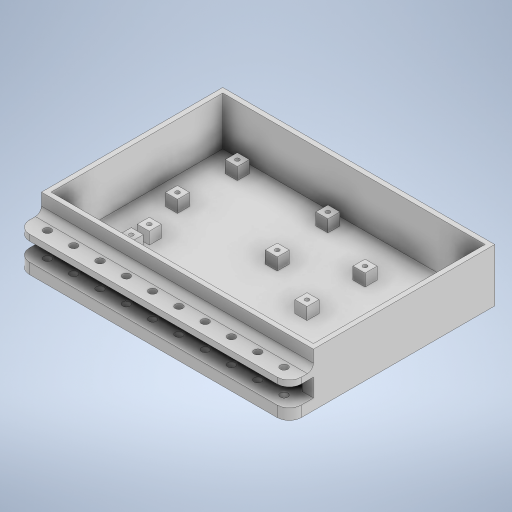
# Autodesk Inventor part: ebox
Saved by Autodesk Inventor 2024.3 (Build 283343000, 343)
## iProperties
Created: 2025-01-01
Part Number: ebox
Material: Generic
Document SubType Name: Modeling
Designer: email
Density: 1 g/cm^3
Appearance: Default
Author: email
Autodesk Inventor part; units mm, degrees
ref_plane "YZ Plane" through (0, 0, 0) normal (1, 0, 0) x (0, 1, 0)
ref_plane "XZ Plane" through (0, 0, 0) normal (0, 1, 0) x (-1, 0, 0)
ref_plane "XY Plane" through (0, 0, 0) normal (0, 0, 1) x (1, 0, 0)
sketch "Sketch1" plane through (0, 0, 0) normal (0, 1, 0) x (-1, 0, 0)
  line L0 (0, 0) -> (-225, 0)
  line L1 (-225, 0) -> (-225, -150)
  line L2 (-225, -150) -> (0, -150)
  line L3 (0, -150) -> (0, 0)
  line L4 (-12.5, -136.845) -> (-114.1, -136.845)
  line L5 (-114.1, -136.845) -> (-114.1, -83.505)
  line L6 (-114.1, -83.505) -> (-12.5, -83.505)
  line L7 (-12.5, -83.505) -> (-12.5, -136.845)
  line L8 (-4, -4) -> (-221, -4)
  line L9 (-221, -4) -> (-221, -146)
  line L10 (-221, -146) -> (-4, -146)
  line L11 (-4, -146) -> (-4, -4)
  line L12 (-153.3391, -114.3444) -> (-208.3391, -114.3444)
  line L13 (-208.3391, -114.3444) -> (-208.3391, -59.3444)
  line L14 (-208.3391, -59.3444) -> (-153.3391, -59.3444)
  line L15 (-153.3391, -59.3444) -> (-153.3391, -114.3444)
  line L16 (-12.6469, -54.1694) -> (-42.6469, -54.1694)
  line L17 (-42.6469, -54.1694) -> (-42.6469, -34.1694)
  line L18 (-42.6469, -34.1694) -> (-12.6469, -34.1694)
  line L19 (-12.6469, -34.1694) -> (-12.6469, -54.1694)
  line L20 (-15.41, -128.945) -> (-4, -128.945)
  line L21 (-4, -128.945) -> (-4, -117.045)
  line L22 (-4, -117.045) -> (-15.41, -117.045)
  line L23 (-15.41, -117.045) -> (-15.41, -128.945)
  circle A0 centre (-27.74, -134.305) radius 1.75
  circle A1 centre (-26.47, -86.045) radius 1.75
  circle A2 centre (-102.67, -134.305) radius 1.75
  circle A3 centre (-109.02, -86.045) radius 1.75
  circle A4 centre (-156.8391, -110.8444) radius 1.75
  circle A5 centre (-204.8391, -110.8444) radius 1.75
  circle A6 centre (-156.8391, -62.8444) radius 1.75
  circle A7 centre (-204.8391, -62.8444) radius 1.75
  circle A8 centre (-37.5669, -51.6294) radius 1.75
  circle A9 centre (-37.5669, -36.7094) radius 1.75
  line L24 (-22.74, -139.305) -> (-32.74, -139.305)
  line L25 (-32.74, -139.305) -> (-32.74, -129.305)
  line L26 (-32.74, -129.305) -> (-22.74, -129.305)
  line L27 (-22.74, -129.305) -> (-22.74, -139.305)
  line L28 (-22.74, -139.305) -> (-32.74, -129.305) construction
  line L29 (-32.74, -139.305) -> (-22.74, -129.305) construction
  line L30 (-21.47, -81.045) -> (-31.47, -81.045)
  line L31 (-31.47, -81.045) -> (-31.47, -91.045)
  line L32 (-31.47, -91.045) -> (-21.47, -91.045)
  line L33 (-21.47, -91.045) -> (-21.47, -81.045)
  line L34 (-21.47, -81.045) -> (-31.47, -91.045) construction
  line L35 (-31.47, -81.045) -> (-21.47, -91.045) construction
  line L36 (-114.02, -81.045) -> (-104.02, -81.045)
  line L37 (-104.02, -81.045) -> (-104.02, -91.045)
  line L38 (-104.02, -91.045) -> (-114.02, -91.045)
  line L39 (-114.02, -91.045) -> (-114.02, -81.045)
  line L40 (-114.02, -81.045) -> (-104.02, -91.045) construction
  line L41 (-104.02, -81.045) -> (-114.02, -91.045) construction
  line L42 (-107.67, -139.305) -> (-97.67, -139.305)
  line L43 (-97.67, -139.305) -> (-97.67, -129.305)
  line L44 (-97.67, -129.305) -> (-107.67, -129.305)
  line L45 (-107.67, -129.305) -> (-107.67, -139.305)
  line L46 (-107.67, -139.305) -> (-97.67, -129.305) construction
  line L47 (-97.67, -139.305) -> (-107.67, -129.305) construction
  line L48 (-151.8391, -115.8444) -> (-161.8391, -115.8444)
  line L49 (-161.8391, -115.8444) -> (-161.8391, -105.8444)
  line L50 (-161.8391, -105.8444) -> (-151.8391, -105.8444)
  line L51 (-151.8391, -105.8444) -> (-151.8391, -115.8444)
  line L52 (-151.8391, -115.8444) -> (-161.8391, -105.8444) construction
  line L53 (-161.8391, -115.8444) -> (-151.8391, -105.8444) construction
  line L54 (-209.8391, -115.8444) -> (-199.8391, -115.8444)
  line L55 (-199.8391, -115.8444) -> (-199.8391, -105.8444)
  line L56 (-199.8391, -105.8444) -> (-209.8391, -105.8444)
  line L57 (-209.8391, -105.8444) -> (-209.8391, -115.8444)
  line L58 (-209.8391, -115.8444) -> (-199.8391, -105.8444) construction
  line L59 (-199.8391, -115.8444) -> (-209.8391, -105.8444) construction
  line L60 (-209.8391, -57.8444) -> (-199.8391, -57.8444)
  line L61 (-199.8391, -57.8444) -> (-199.8391, -67.8444)
  line L62 (-199.8391, -67.8444) -> (-209.8391, -67.8444)
  line L63 (-209.8391, -67.8444) -> (-209.8391, -57.8444)
  line L64 (-209.8391, -57.8444) -> (-199.8391, -67.8444) construction
  line L65 (-199.8391, -57.8444) -> (-209.8391, -67.8444) construction
  line L66 (-161.8391, -57.8444) -> (-151.8391, -57.8444)
  line L67 (-151.8391, -57.8444) -> (-151.8391, -67.8444)
  line L68 (-151.8391, -67.8444) -> (-161.8391, -67.8444)
  line L69 (-161.8391, -67.8444) -> (-161.8391, -57.8444)
  line L70 (-161.8391, -57.8444) -> (-151.8391, -67.8444) construction
  line L71 (-151.8391, -57.8444) -> (-161.8391, -67.8444) construction
  line L72 (-42.5669, -46.6294) -> (-32.5669, -46.6294)
  line L73 (-32.5669, -46.6294) -> (-32.5669, -56.6294)
  line L74 (-32.5669, -56.6294) -> (-42.5669, -56.6294)
  line L75 (-42.5669, -56.6294) -> (-42.5669, -46.6294)
  line L76 (-42.5669, -46.6294) -> (-32.5669, -56.6294) construction
  line L77 (-32.5669, -46.6294) -> (-42.5669, -56.6294) construction
  line L78 (-32.5669, -41.7094) -> (-42.5669, -41.7094)
  line L79 (-42.5669, -41.7094) -> (-42.5669, -31.7094)
  line L80 (-42.5669, -31.7094) -> (-32.5669, -31.7094)
  line L81 (-32.5669, -31.7094) -> (-32.5669, -41.7094)
  line L82 (-32.5669, -41.7094) -> (-42.5669, -31.7094) construction
  line L83 (-42.5669, -41.7094) -> (-32.5669, -31.7094) construction
  line L84 (0, -4) -> (-225, -4)
  line L85 (-225, -4) -> (-225, 20)
  line L86 (-225, 20) -> (0, 20)
  line L87 (0, 20) -> (0, -4)
  circle A10 centre (-15, 10) radius 3.125
  circle A11 centre (-36.75, 10) radius 3.125
  circle A12 centre (-58.5, 10) radius 3.125
  circle A13 centre (-80.25, 10) radius 3.125
  circle A14 centre (-102, 10) radius 3.125
  circle A15 centre (-123.75, 10) radius 3.125
  circle A16 centre (-145.5, 10) radius 3.125
  circle A17 centre (-167.25, 10) radius 3.125
  circle A18 centre (-189, 10) radius 3.125
  circle A19 centre (-210.75, 10) radius 3.125
  point P0 (-156.8391, -62.8444)
  dimension "d0" = 225
  dimension "d1" = 150
  dimension "d2" = 101.6
  dimension "d3" = 53.34
  dimension "d5" = 4
  dimension "d6" = 217
  dimension "d7" = 142
  dimension "d8" = 4
  dimension "d9" = 8.5
  dimension "d10" = 55
  dimension "d11" = 55
  dimension "d12" = 30
  dimension "d13" = 20
  dimension "d14" = 7.9
  dimension "d15" = 8.5
  dimension "d16" = 11.9
  dimension "d17" = 2.54
  dimension "d18" = 3.5
  dimension "d19" = 15.24
  dimension "d20" = 3.5
  dimension "d21" = 3.5
  dimension "d22" = 3.5
  dimension "d23" = 2.54
  dimension "d24" = 13.97
  dimension "d26" = 2.54
  dimension "d27" = 90.17
  dimension "d28" = 2.54
  dimension "d29" = 96.52
  dimension "d30" = 3.5
  dimension "d31" = 3.5
  dimension "d32" = 3.5
  dimension "d33" = 3.5
  dimension "d34" = 3.5
  dimension "d35" = 3.5
  dimension "d36" = 3.5
  dimension "d38" = 3.5
  dimension "d39" = 3.5
  dimension "d40" = 3.5
  dimension "d41" = 3.5
  dimension "d42" = 3.5
  dimension "d43" = 3.5
  dimension "d44" = 2.54
  dimension "d45" = 5.08
  dimension "d46" = 5.08
  dimension "d47" = 2.54
  dimension "d54" = 10
  dimension "d55" = 10
  dimension "d56" = 10
  dimension "d57" = 10
  dimension "d58" = 10
  dimension "d59" = 10
  dimension "d60" = 10
  dimension "d61" = 10
  dimension "d65" = 10
  dimension "d66" = 10
  dimension "d67" = 10
  dimension "d68" = 10
  dimension "d69" = 10
  dimension "d70" = 10
  dimension "d71" = 10
  dimension "d72" = 10
  dimension "d73" = 10
  dimension "d74" = 10
  dimension "d75" = 10
  constraints: 176 end point, 34 parallel, 21 midpoint, 20 centre point, 18 horizontal, 17 perpendicular, 2 point on line, 18 other
  measures "d0" distance of L1.end L2.end
  measures "d1" distance of L0.end L1.end
  measures "d2" distance of L4.start L4.end
  measures "d3" distance of L4.end L5.end
  measures "d5" distance between parallel lines of L0 L8
  measures "d6" distance of L9.end L10.end
  measures "d7" distance of L8.end L9.end
  measures "d8" distance between parallel lines of L3 L11
  measures "d9" distance between parallel lines of L11 L7
  measures "d10" distance of L12.end L13.end
  measures "d11" distance of L13.end L14.end
  measures "d12" distance of L16.start L16.end
  measures "d13" distance of L16.end L17.end
  measures "d14" distance between parallel lines of L4 L20
  measures "d15" distance between parallel lines of L7 L21
  measures "d16" distance of L22.end L20.start
  measures "d17" distance from line of L4 A0.centre
  measures "d18" diameter of A0
  measures "d19" distance from line of L7 A0.centre
  measures "d20" diameter of A1
  measures "d21" diameter of A3
  measures "d22" diameter of A2
  measures "d23" distance from line of L6 A1.centre
  measures "d24" distance from line of L7 A1.centre
  measures "d26" distance from line of L4 A2.centre
  measures "d27" distance from line of A2.centre L7
  measures "d28" distance from line of L6 A3.centre
  measures "d29" distance from line of L7 A3.centre
  measures "d30" diameter of A4
  measures "d31" diameter of A5
  measures "d32" diameter of A6
  measures "d33" diameter of A7
  measures "d34" distance from line of L12 A4.centre
  measures "d35" distance from line of L15 A4.centre
  measures "d36" distance from line of L14 A6.centre
  measures "d38" distance from line of L13 A7.centre
  measures "d39" distance from line of L14 A7.centre
  measures "d40" distance from line of L13 A5.centre
  measures "d41" distance from line of L12 A5.centre
  measures "d42" diameter of A8
  measures "d43" diameter of A9
  measures "d44" distance from line of L16 A8.centre
  measures "d45" distance from line of L17 A8.centre
  measures "d46" distance from line of L17 A9.centre
  measures "d47" distance from line of L18 A9.centre
  measures "d54" distance of L24.end L25.end
  measures "d55" distance of L25.end L26.end
  measures "d56" distance of L42.end L43.end
  measures "d57" distance of L43.end L44.end
  measures "d58" distance of L31.end L32.end
  measures "d59" distance of L30.end L31.end
  measures "d60" distance of L37.end L38.end
  measures "d61" distance of L36.end L37.end
  measures "d65" distance of L48.end L49.end
  measures "d66" distance of L49.end L50.end
  measures "d67" distance of L54.end L55.end
  measures "d68" distance of L55.end L56.end
  measures "d69" distance of L66.end L67.end
  measures "d70" distance of L66.start L66.end
  measures "d71" distance of L62.end L60.start
  measures "d72" distance of L60.start L60.end
  measures "d73" distance of L73.end L74.end
  measures "d74" distance of L72.end L73.end
  measures "d75" distance of L78.start L78.end
extrude "Extrusion1" add sketch "Sketch1" against normal blind 4 contours L3 L84 L8 L1 L0 | L3 L2 L1 L84 L9 L10 L11 | L11 L22 L7 L6 L33 L30 L31 L37 L36 L39 L5 L4 L45 L42 L43 L25 L24 L27 L20 L10 L9 L8 | L11 L20 L7 L22 | L22 L23 L20 L7 L4 L27 L26 L25 L43 L44 L45 L5 L6 L39 L38 L37 L31 L32 L33 | L7 L20 L23 L22 | L33 L32 L31 L6 | L6 L31 L30 L33 | L27 L24 L25 L4 | L4 L25 L26 L27 | L37 L38 L39 L6 | L6 L39 L36 L37 | L43 L42 L45 L4 | L4 L45 L44 L43 | L15 L50 L51 L48 L49 L12 | L12 L49 L50 L15 | L12 L55 L56 L13 L62 L61 L14 L69 L68 L15 L50 L49 | L55 L54 L57 L56 L13 L12 | L12 L13 L56 L55 | L68 L69 L14 L15 | L15 L14 L69 L66 L67 L68 | L62 L63 L60 L61 L14 L13 | L13 L14 L61 L62 | L16 L73 L72 L75 L17 L18 L79 L78 L81 L19 | L73 L74 L75 L16 | L16 L75 L72 L73 | L81 L78 L79 L18 | L18 L79 L80 L81 | A0 | A1 | A2 | A3 | A4 | A5 | A6 | A7 | A8 | A9
extrude "Extrusion2" add sketch "Sketch1" along normal blind 40 contours L3 L84 L8 L1 L0 | L3 L2 L1 L84 L9 L10 L11
extrude "Extrusion3" add sketch "Sketch1" along normal blind 10 contours L33 L32 L31 L6 | L6 L31 L30 L33 | L27 L24 L25 L4 | L4 L25 L26 L27 | L37 L38 L39 L6 | L6 L39 L36 L37 | L43 L42 L45 L4 | L4 L45 L44 L43 | L15 L50 L51 L48 L49 L12 | L12 L49 L50 L15 | L55 L54 L57 L56 L13 L12 | L12 L13 L56 L55 | L68 L69 L14 L15 | L15 L14 L69 L66 L67 L68 | L62 L63 L60 L61 L14 L13 | L13 L14 L61 L62 | L73 L74 L75 L16 | L16 L75 L72 L73 | L81 L78 L79 L18 | L18 L79 L80 L81
extrude "Extrusion4" add sketch "Sketch1" along normal blind 5 and the other way blind 4 contours L0 L85 L86 L87
sketch "Sketch2" plane through (0, 40, 0) normal (0, 0, 1) x (1, 0, 0)
  line L0 (10, -20) -> (20, -20)
  line L1 (20, -20) -> (20, -35)
  line L2 (20, -35) -> (10, -35)
  line L3 (10, -35) -> (10, -20)
  line L4 (10, -20) -> (20, -35) construction
  line L5 (20, -20) -> (10, -35) construction
  line L6 (31.75, -20) -> (41.75, -20)
  line L7 (41.75, -20) -> (41.75, -35)
  line L8 (41.75, -35) -> (31.75, -35)
  line L9 (31.75, -35) -> (31.75, -20)
  line L10 (31.75, -20) -> (41.75, -35) construction
  line L11 (41.75, -20) -> (31.75, -35) construction
  line L12 (53.5, -20) -> (63.5, -20)
  line L13 (63.5, -20) -> (63.5, -35)
  line L14 (63.5, -35) -> (53.5, -35)
  line L15 (53.5, -35) -> (53.5, -20)
  line L16 (53.5, -20) -> (63.5, -35) construction
  line L17 (63.5, -20) -> (53.5, -35) construction
  line L18 (75.25, -20) -> (85.25, -20)
  line L19 (85.25, -20) -> (85.25, -35)
  line L20 (85.25, -35) -> (75.25, -35)
  line L21 (75.25, -35) -> (75.25, -20)
  line L22 (75.25, -20) -> (85.25, -35) construction
  line L23 (85.25, -20) -> (75.25, -35) construction
  line L24 (97, -20) -> (107, -20)
  line L25 (107, -20) -> (107, -35)
  line L26 (107, -35) -> (97, -35)
  line L27 (97, -35) -> (97, -20)
  line L28 (97, -20) -> (107, -35) construction
  line L29 (107, -20) -> (97, -35) construction
  line L30 (118.75, -20) -> (128.75, -20)
  line L31 (128.75, -20) -> (128.75, -35)
  line L32 (128.75, -35) -> (118.75, -35)
  line L33 (118.75, -35) -> (118.75, -20)
  line L34 (118.75, -20) -> (128.75, -35) construction
  line L35 (128.75, -20) -> (118.75, -35) construction
  line L36 (140.5, -20) -> (150.5, -20)
  line L37 (150.5, -20) -> (150.5, -35)
  line L38 (150.5, -35) -> (140.5, -35)
  line L39 (140.5, -35) -> (140.5, -20)
  line L40 (140.5, -20) -> (150.5, -35) construction
  line L41 (150.5, -20) -> (140.5, -35) construction
  line L42 (162.25, -20) -> (172.25, -20)
  line L43 (172.25, -20) -> (172.25, -35)
  line L44 (172.25, -35) -> (162.25, -35)
  line L45 (162.25, -35) -> (162.25, -20)
  line L46 (162.25, -20) -> (172.25, -35) construction
  line L47 (172.25, -20) -> (162.25, -35) construction
  line L48 (184, -20) -> (194, -20)
  line L49 (194, -20) -> (194, -35)
  line L50 (194, -35) -> (184, -35)
  line L51 (184, -35) -> (184, -20)
  line L52 (184, -20) -> (194, -35) construction
  line L53 (194, -20) -> (184, -35) construction
  line L54 (205.75, -20) -> (215.75, -20)
  line L55 (215.75, -20) -> (215.75, -35)
  line L56 (215.75, -35) -> (205.75, -35)
  line L57 (205.75, -35) -> (205.75, -20)
  line L58 (205.75, -20) -> (215.75, -35) construction
  line L59 (215.75, -20) -> (205.75, -35) construction
  line L60 (0, -35) -> (0, 0) projected
  line L61 (0, -35) -> (225, -35) projected
  point P0 (15, -27.5)
  point P1 (36.75, -27.5)
  point P2 (58.5, -27.5)
  point P3 (80.25, -27.5)
  point P4 (102, -27.5)
  point P5 (123.75, -27.5)
  point P6 (145.5, -27.5)
  point P7 (167.25, -27.5)
  point P8 (189, -27.5)
  point P9 (210.75, -27.5)
  dimension "d105" = 10
  dimension "d106" = 15
  dimension "d109" = 21.75
  dimension "d132" = 15
  dimension "d133" = 7.5
  constraints: 120 end point, 20 midpoint, 2 horizontal, 2 parallel, 1 collinear, 1 perpendicular, 98 other
  measures "d105" distance of L0.start L0.end
  measures "d106" distance of L2.end L0.start
  measures "d109" distance of L0.start L6.start
  measures "d132" distance from line of L60 point (15, -27.5)
  measures "d133" distance from line of L61 point (15, -27.5)
extrude "Extrusion5" cut sketch "Sketch2" against normal blind 4
ref_plane "Work Plane1" through (0, 20, 0) normal (0, 1, 0) x (1, 0, 0)
sketch "Sketch3" plane through (0, 20, 0) normal (0, 1, 0) x (1, 0, 0)
  line L0 (0, 150) -> (0, 0) projected
  line L1 (0, 0) -> (225, 0)
  line L2 (225, 0) -> (225, -20)
  line L3 (225, -20) -> (0, -20)
  line L4 (0, -20) -> (0, 0)
  circle A0 centre (15, -10) radius 3.125 projected
  circle A1 centre (15, -10) radius 3.125
  circle A2 centre (36.75, -10) radius 3.125
  circle A3 centre (58.5, -10) radius 3.125
  circle A4 centre (80.25, -10) radius 3.125
  circle A5 centre (102, -10) radius 3.125
  circle A6 centre (123.75, -10) radius 3.125
  circle A7 centre (145.5, -10) radius 3.125
  circle A8 centre (167.25, -10) radius 3.125
  circle A9 centre (189, -10) radius 3.125
  circle A10 centre (210.75, -10) radius 3.125
  dimension "d118" = 20
  dimension "d119" = 225
  dimension "d120" = 6.25
  dimension "d121" = 15
  dimension "d122" = 10
  dimension "d125" = 21.75
  constraints: 10 centre point, 8 end point, 2 horizontal, 2 parallel, 1 coincident, 1 perpendicular, 18 other
  measures "d118" distance of L1.end L2.end
  measures "d119" distance of L2.end L3.end
  measures "d120" diameter of A1
  measures "d121" distance from line of L4 A1.centre
  measures "d122" distance from line of L1 A1.centre
  measures "d125" distance of A1.centre A2.centre
extrude "Extrusion6" add sketch "Sketch3" along normal blind 5
fillet "Fillet2" radius 10 4 edges at (0, 22.5, 20) (0, 0.5, 20) (225, 22.5, 20) (225, 0.5, 20)
fillet "Fillet3" radius 5 1 edges at (112.5, 25, 0)
body "Solid1"
